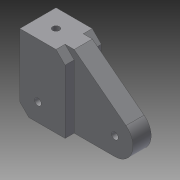
# Autodesk Inventor part: Finger Joint
Saved by Autodesk Inventor 2014 SP1 (Build 180222100, 222)
## iProperties
Created: 2014-01-25
Part Number: Finger Joint
Material: Generic
Document SubType Name: Modeling
Designer: tom
Density: 1 g/cm^3
Appearance: Default
Author: tom
Autodesk Inventor part; units mm, degrees
ref_plane "YZ Plane" through (0, 0, 0) normal (1, 0, 0) x (0, 1, 0)
ref_plane "XZ Plane" through (0, 0, 0) normal (0, 1, 0) x (-1, 0, 0)
ref_plane "XY Plane" through (0, 0, 0) normal (0, 0, 1) x (1, 0, 0)
sketch "Sketch1" plane through (0, 0, 0) normal (0, 0, 1) x (1, 0, 0)
  circle A0 centre (9.5, 5) radius 0.75
  arc A1 (9.5, 1) -> (11.9441, 8.1664) centre (9.5, 5) ccw
  circle A2 centre (9.5, 5) radius 6.5 construction
  line L0 (9.5, 5) -> (-5.5, 5) construction
  circle A3 centre (-5.5, 5) radius 0.75
  line L1 (9.5, 1) -> (-9.5, 1)
  line L2 (-9.5, 1) -> (-9.5, 9)
  line L3 (-9.5, 9) -> (-9.5, 17)
  line L4 (-9.5, 17) -> (0.5, 17)
  line L5 (0.5, 17) -> (11.9441, 8.1664)
  point P0 (0, 0)
  dimension "d0" = 8
  dimension "d1" = 13
  dimension "d4" = 1.5
  dimension "d19" = 8
  dimension "d20" = 10
  dimension "d37" = 19
  dimension "d39" = 4
  constraints: 12 end point, 4 centre point, 2 coincident, 2 perpendicular, 2 point on circle, 2 tangent, 1 horizontal, 1 parallel
  measures "d0" diameter of A1
  measures "d1" diameter of A2
  measures "d4" diameter of A3
  measures "d19" distance of L2.end L3.end
  measures "d20" distance of L3.end L4.end
  measures "d37" distance of L1.start L1.end
  measures "d39" distance from line of L2 L0.end
extrude "Extrusion1" add sketch "Sketch1" along normal blind 4
sketch "Sketch5" plane through (-9.5, 17, 0) normal (0, 1, 0) x (1, 0, 0)
  line L0 (10, 0) -> (0, 0) projected
  line L1 (0, 0) -> (0, -4) projected
  line L2 (10, -4) -> (0, -4) projected
  line L3 (10, 0) -> (10, -4) projected
  line L4 (0, 2) -> (10, 2)
  line L5 (10, 2) -> (10, -6)
  line L6 (10, -6) -> (0, -6)
  line L7 (0, -6) -> (0, 2)
  point P0 (9.5, 0)
  dimension "d40" = 2
  dimension "d41" = 8
  dimension "d42" = 10
  constraints: 8 end point, 2 parallel, 1 horizontal, 1 perpendicular
  measures "d40" distance between parallel lines of L4 L0
  measures "d41" distance of L6.end L4.start
  measures "d42" distance of L5.end L6.end
extrude "Extrusion5" add sketch "Sketch5" against normal blind 16 contours L0 L7 L4 L5 | L5 L6 L7 L2
sketch "Sketch6" plane through (9.5, 1, 0) normal (0, -1, 0) x (1, 0, 0)
  line L0 (-9, 6) -> (-19, 6) projected
  line L1 (-19, 6) -> (-19, -2) projected
  line L2 (-19, -2) -> (-9, -2) projected
  line L3 (-9, -2) -> (-9, 0) projected
  line L4 (-19, 4) -> (-11, 4)
  line L5 (-11, 4) -> (-11, 0)
  line L6 (-11, 0) -> (-19, 0)
  point P0 (-9.5, 0)
  dimension "d45" = 2
  dimension "d46" = 2
  dimension "d47" = 8
  constraints: 6 end point, 3 perpendicular, 2 point on line
  measures "d45" distance between parallel lines of L0 L4
  measures "d46" distance between parallel lines of L2 L6
  measures "d47" distance between parallel lines of L1 L5
extrude "Extrusion6" cut sketch "Sketch6" against normal blind 8
chamfer "Chamfer5" distance 2 angle 45 4 edges at (-9.5, 1, 5) (-9.5, 1, -1) (0.5, 17, 5) (0.5, 17, -1)
sketch "Sketch7" plane through (0.5, 17, 4) normal (0, 1, 0) x (1, 0, 0)
  line L0 (-10, 6) -> (-2, 6) projected
  line L1 (0, 4) -> (0, 0) projected
  circle A0 centre (-6, 2) radius 0.75
  point P0 (-8, 6)
  point P1 (-0.5, 4)
  dimension "d53" = 1.5
  dimension "d54" = 4
  dimension "d55" = 6
  constraints: 1 centre point
  measures "d53" diameter of A0
  measures "d54" distance from line of A0.centre L0
  measures "d55" distance from line of L1 A0.centre
extrude "Extrusion7" cut sketch "Sketch7" against normal blind 6
sketch "Sketch8" plane through (-9.5, 17, 6) normal (0, 0, 1) x (1, 0, 0)
  line L0 (0, 0) -> (0, -14) projected
  line L1 (10, -16) -> (2, -16) projected
  circle A0 centre (4, -12) radius 0.75
  point P0 (9.5, -17)
  dimension "d58" = 1.5
  dimension "d59" = 4
  dimension "d60" = 4
  constraints: 1 centre point
  measures "d58" diameter of A0
  measures "d59" distance from line of L0 A0.centre
  measures "d60" distance from line of L1 A0.centre
extrude "Extrusion8" cut sketch "Sketch8" against normal blind 8
body "Solid1"
